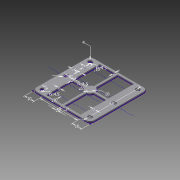
# Autodesk Inventor part: MechBottomPlate
Saved by Autodesk Inventor 2014 SP1 (Build 180222100, 222)
## iProperties
Created: 2015-03-02
Part Number: MechBottomPlate
Material: Generic
Document SubType Name: Modeling
Designer: Erin
Density: 1 g/cm^3
Appearance: Default
Author: Erin
Autodesk Inventor part; units mm, degrees
ref_plane "YZ Plane" through (0, 0, 0) normal (1, 0, 0) x (0, 1, 0)
ref_plane "XZ Plane" through (0, 0, 0) normal (0, 1, 0) x (-1, 0, 0)
ref_plane "XY Plane" through (0, 0, 0) normal (0, 0, 1) x (1, 0, 0)
sketch "Sketch1" plane through (0, 0, 0) normal (0, 0, 1) x (1, 0, 0)
  line L0 (-20, 30) -> (20, 30)
  line L1 (20, 30) -> (20, -30)
  line L2 (20, -30) -> (-20, -30)
  line L3 (-20, -30) -> (-20, 30)
  line L4 (-20, 30) -> (-26, 30)
  line L5 (-30, 26) -> (-30, -26)
  line L6 (-26, -30) -> (-20, -30)
  line L7 (-20, -30) -> (-20, 30)
  line L8 (20, 30) -> (26, 30)
  line L9 (30, 26) -> (30, -26)
  line L10 (26, -30) -> (20, -30)
  line L11 (20, -30) -> (20, 30)
  line L12 (-43.9092, 0) -> (47.176, 0) construction
  circle A0 centre (-25, 0) radius 2.25
  line L13 (-30, 20) -> (30, 20) construction
  circle A1 centre (-25, 25) radius 2.25
  line L14 (-30, -20) -> (30, -20) construction
  circle A2 centre (-25, -25) radius 2.25
  line L15 (-30, 5) -> (30, 5) construction
  line L16 (-30, -5) -> (30, -5) construction
  line L17 (-28, 18) -> (-22, 18)
  line L18 (-22, 18) -> (-22, 7)
  line L19 (-22, 7) -> (-28, 7)
  line L20 (-28, 7) -> (-28, 18)
  line L21 (-18, 28) -> (18, 28)
  line L22 (18, 28) -> (18, -28)
  line L23 (18, -28) -> (-18, -28)
  line L24 (-18, -28) -> (-18, 28)
  line L25 (-18, 1) -> (18, 1)
  line L26 (18, 1) -> (18, -1)
  line L27 (18, -1) -> (-18, -1)
  line L28 (-18, -1) -> (-18, 1)
  line L29 (-1, 28) -> (1, 28)
  line L30 (1, 28) -> (1, -28)
  line L31 (1, -28) -> (-1, -28)
  line L32 (-1, -28) -> (-1, 28)
  arc A3 (-26, 30) -> (-30, 26) centre (-26, 26) ccw
  arc A4 (-30, -26) -> (-26, -30) centre (-26, -26) ccw
  arc A5 (26, -30) -> (30, -26) centre (26, -26) ccw
  arc A6 (30, 26) -> (26, 30) centre (26, 26) ccw
  circle A7 centre (0, 0) radius 5
  point P0 (0, 30)
  point P1 (20, 0)
  point P2 (-30, -30)
  point P3 (30, -30)
  point P4 (-18, 0)
  point P5 (0, 28)
  dimension "d0" = 40
  dimension "d1" = 60
  dimension "d2" = 10
  dimension "d3" = 10
  dimension "d4" = 4.5
  dimension "d5" = 10
  dimension "d6" = 4.5
  dimension "d7" = 5
  dimension "d8" = 4.5
  dimension "d9" = 5
  dimension "d10" = 5
  dimension "d11" = 5
  dimension "d12" = 5
  dimension "d13" = 10
  dimension "d14" = 5
  dimension "d15" = 5
  dimension "d16" = 2
  dimension "d17" = 2
  dimension "d18" = 2
  dimension "d19" = 2
  dimension "d20" = 2
  dimension "d21" = 2
  dimension "d22" = 2
  dimension "d23" = 2
  dimension "d24" = 2
  dimension "d25" = 2
  dimension "d26" = 4
  dimension "d33" = 10
  constraints: 66 end point, 17 point on line, 14 parallel, 12 perpendicular, 8 centre point, 8 horizontal, 8 point on circle, 8 tangent, 4 midpoint, 3 equal radius, 2 collinear, 2 horizontal alignment, 2 vertical alignment, 1 coincident
  measures "d0" distance of L1.end L2.end
  measures "d1" distance of L0.end L1.end
  measures "d2" distance of L6.end point (-30, -30)
  measures "d3" distance of point (30, -30) L10.end
  measures "d4" diameter of A0
  measures "d5" distance between parallel lines of L13 L0
  measures "d6" diameter of A1
  measures "d7" distance from line of A1.centre L13
  measures "d8" diameter of A2
  measures "d9" distance from line of A2.centre L14
  measures "d10" distance from line of A2.centre L5
  measures "d11" distance from line of A1.centre L5
  measures "d12" distance from line of A0.centre L5
  measures "d13" distance between parallel lines of L2 L14
  measures "d14" distance between parallel lines of L12 L15
  measures "d15" distance between parallel lines of L16 L12
  measures "d16" distance between parallel lines of L17 L13
  measures "d17" distance between parallel lines of L5 L20
  measures "d18" distance between parallel lines of L18 L3
  measures "d19" distance between parallel lines of L19 L15
  measures "d20" distance between parallel lines of L2 L23
  measures "d21" distance between parallel lines of L24 L3
  measures "d22" distance between parallel lines of L1 L22
  measures "d23" distance between parallel lines of L21 L0
  measures "d24" distance of L27.end L25.start
  measures "d25" distance of L30.end L31.end
  measures "d26" radius of A3
  measures "d33" diameter of A7
extrude "Extrusion1" add sketch "Sketch1" along normal blind 1.5 contours L0 L1 L2 L3 | L3 L6 A4 L5 A3 L4 | L8 A6 L9 A5 L10 L1 | A0 | A1 | A2 | L17 L18 L19 L20 | L21 L30 A7 L32 | L25 A7 L27 L24 | A7 L30 L25 L32 | L32 L25 A7 | L25 L32 L27 A7 | A7 L25 L30 | L25 L30 L27 L32 | L27 L32 A7 | L22 L27 A7 L25 | L25 A7 L27 L30 | L27 L30 A7 L32 | L32 A7 L30 L23 | L27 A7 L30
extrude "Extrusion2" cut sketch "Sketch1" along normal blind 2 contours A0 | A1 | A2
mirror "Mirror2" about plane through (0, 0, 0) normal (1, 0, 0) of "Extrusion2"
equation "\"d4\" = screw"
equation "\"d6\" = screw"
equation "\"d8\" = screw"
equation "\"screw\" = 4.5"
body "Solid1"
